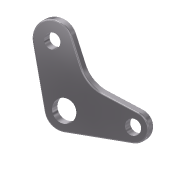
# Autodesk Inventor part: Bracket - Optimization - Copy
Saved by Autodesk Inventor 2020.1 (Build 241239000, 239)
## iProperties
Part Number: Bracket - Optimization - Copy
Document SubType Name: Modeling
Created: 2003-07-06
Designer: Ronald Myers
Manufacturer: Standard
Standards Organization: Custom
Stock Number: WeldExer_base
Density: 2.7 g/cm^3
Material: Aluminum 6061
Appearance: Aluminum (Polished)
Control State: 0
Master: False
Checked Out: False
Shininess: 64.0
Length Units: 11269
Angle Units: 11279
Time Units: 11290
Mass Units: 11286
Length Display Precision: 3
Angle Display Precision: 2
Compacted: True
Density: 0.0
Volumn: 0.0
Area: 0.0
PropertySet Name: Model Information
Author: Ronald Myers
Autodesk Inventor part; units mm, degrees
ref_plane "YZ Plane" through (0, 0, 0) normal (1, 0, 0) x (0, 1, 0)
ref_plane "XZ Plane" through (0, 0, 0) normal (0, 1, 0) x (-1, 0, 0)
ref_plane "XY Plane" through (0, 0, 0) normal (0, 0, 1) x (1, 0, 0)
sketch "Sketch1" plane through (0, 0, 0) normal (0, 0, 1) x (1, 0, 0)
  arc A0 (-36.3497, -18.0713) -> (-15.9827, -32.4309) centre (-25.5909, -24.4351) ccw
  arc A1 (35.8842, -10.6617) -> (38.9651, 7.8249) centre (35.8842, -1.1617) ccw
  arc A2 (-1.287, 21.6247) -> (-16.0996, 16.1641) centre (-5.3408, 9.8003) ccw
  arc A3 (12.4467, -10.6617) -> (-4.4637, -18.5891) centre (12.4467, -32.6617) ccw
  line L0 (-15.9827, -32.4309) -> (-4.4637, -18.5891)
  line L1 (12.4467, -10.6617) -> (35.8842, -10.6617)
  line L2 (38.9651, 7.8249) -> (-1.287, 21.6247)
  line L3 (-16.0996, 16.1641) -> (-36.3497, -18.0713)
  dimension "d0" = 12.5
  dimension "d1" = 9.5
  dimension "d2" = 12.5
  dimension "d3" = 22
  constraints: 8 end point, 8 point on circle, 8 tangent, 4 centre point, 1 horizontal
  measures "d0" radius of A0
  measures "d1" radius of A1
  measures "d2" radius of A2
  measures "d3" radius of A3
extrude "Extrusion1" add sketch "Sketch1" along normal mid plane 6.5
sketch "Sketch2" plane through (0, 0, 3.25) normal (0, 0, 1) x (1, 0, 0)
  arc A0 (-36.3497, -18.0713) -> (-15.9827, -32.4309) centre (-25.5909, -24.4351) ccw projected
  arc A1 (-1.287, 21.6247) -> (-16.0996, 16.1641) centre (-5.3408, 9.8003) ccw projected
  arc A2 (35.8842, -10.6617) -> (38.9651, 7.8249) centre (35.8842, -1.1617) ccw projected
  line L0 (-36.3497, -18.0713) -> (-16.0996, 16.1641) projected
  line L1 (-4.4637, -18.5891) -> (-15.9827, -32.4309) projected
  arc A3 (12.4467, -10.6617) -> (-4.4637, -18.5891) centre (12.4467, -32.6617) ccw projected
  line L2 (35.8842, -10.6617) -> (12.4467, -10.6617) projected
  line L3 (-1.287, 21.6247) -> (38.9651, 7.8249) projected
hole "Hole1" at (-25.5909, -24.4351, 3.25) direction (0, 0, -1) diameter 10 end through all
sketch "Sketch3" plane through (0, 0, 3.25) normal (0, 0, 1) x (1, 0, 0)
  arc A0 (-1.287, 21.6247) -> (-16.0996, 16.1641) centre (-5.3408, 9.8003) ccw projected
hole "Hole2" at (-5.3408, 9.8003, 3.25) direction (0, 0, -1) diameter 15 end through all
sketch "Sketch4" plane through (0, 0, 3.25) normal (0, 0, 1) x (1, 0, 0)
  arc A0 (35.8842, -10.6617) -> (38.9651, 7.8249) centre (35.8842, -1.1617) ccw projected
hole "Hole3" at (35.8842, -1.1617, 3.25) direction (0, 0, -1) diameter 10 end through all
fillet "Fillet1" radius 1 16 edges at (18.8391, 14.7248, 3.25) (45.2549, -2.7234, 3.25) (24.1654, -10.6617, 3.25) (3.1086, -12.7419, 3.25) (-10.2232, -25.51, 3.25) (-32.7937, -34.6512, 3.25) (-26.2246, -0.9536, 3.25) (-9.6644, 21.5287, 3.25) (18.8391, 14.7248, -3.25) (-9.6644, 21.5287, -3.25) (-26.2246, -0.9536, -3.25) (-32.7937, -34.6512, -3.25) (-10.2232, -25.51, -3.25) (3.1086, -12.7419, -3.25) (24.1654, -10.6617, -3.25) (45.2549, -2.7234, -3.25)
body "Solid1"
